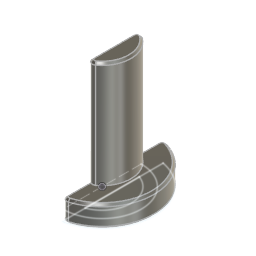
SpoolHanger (Autodesk Fusion 360 design; units mm, degrees)
Autodesk Fusion 360 part; units mm, degrees
note: some values were not read from the file. Chosen so that the rebuilt part matches the saved one: which face or edge a step refers to. Set by a fixed rule: which sketch regions a step uses.
sketch "Sketch1" plane through (0, 0, 0) normal (0, 0, 1) x (1, 0, 0) in component "VerticalArm"
  line L0 (0, 10.4) -> (0, -10.4)
  line L1 (0, 10.4) -> (-131.0205, 10.4)
  line L2 (0, -10.4) -> (-131.0205, -10.4)
  circle A0 centre (-150, 0) radius 21.6421
  line L3 (-139.8, -10.2) -> (-160.2, -10.2)
  line L4 (-160.2, -10.2) -> (-160.2, 10.2)
  line L5 (-160.2, 10.2) -> (-139.8, 10.2)
  line L6 (-139.8, 10.2) -> (-139.8, -10.2)
  line L7 (-139.8, -10.2) -> (-160.2, 10.2) construction
  line L8 (-160.2, -10.2) -> (-139.8, 10.2) construction
  line L9 (-150, 21.6421) -> (-150, -21.6421) construction
  line L10 (-150, 0) -> (0, 0) construction
  point P0 (-150, 0)
  dimension "d137" = 43.2843
  dimension "d138" = 20.4
  dimension "d253" = 20.8
  dimension "d255" = 150
  constraint coincident L10.end origin
  constraint vertical L0
  constraint perpendicular L0 L1
  constraint perpendicular L0 L2
  constraint equal L1 L2
  constraint horizontal L3
  constraint perpendicular L3 L4
  constraint parallel L3 L5
  constraint parallel L4 L6
  constraint coincident L7 P0
  constraint coincident L8 P0
  constraint coincident P0 A0.centre
  constraint equal L4 L5
  constraint midpoint L10.end L0
  constraint vertical L9
  constraint coincident P0 L9
  constraint coincident A0 L9.start
  constraint coincident A0 L9.end
  constraint perpendicular L0 L10
  constraint coincident A0 L1.end
  measures "d137" diameter of A0
  measures "d138" distance of L3.end L4.end
  measures "d253" distance of L0.start L0.end
  measures "d255" distance of L0 L9
sketch "Sketch1 (2)" plane through (0, 0, 0) normal (0, 0, 1) x (1, 0, 0) in component "HorizontalBarInnerPart"
  line L0 (80.8, -9.2) -> (-80.8, -9.2)
  line L1 (-80.8, -9.2) -> (-80.8, 9.2)
  line L2 (-80.8, 9.2) -> (80.8, 9.2)
  line L3 (80.8, 9.2) -> (80.8, -9.2)
  line L4 (80.8, -9.2) -> (-80.8, 9.2) construction
  line L5 (-80.8, -9.2) -> (80.8, 9.2) construction
  arc A0 (-80.8, 9.2) -> (-80.8, -9.2) centre (-80.8, 0) ccw
  arc A1 (-82.4, 7.4297) -> (-82.4, -7.4297) centre (-80.8, 0) ccw
  line L6 (-82.4, -7.4297) -> (-82.4, 7.4297)
  line L7 (0, 9.2) -> (0, -9.2)
  arc A2 (82.4, -7.4297) -> (82.4, 7.4297) centre (80.8, 0) ccw
  arc A3 (80.8, -9.2) -> (80.8, 9.2) centre (80.8, 0) ccw
  line L8 (82.4, -7.4297) -> (82.4, 7.4297)
  dimension "d81" = 161.6
  dimension "d82" = 18.4
  constraint horizontal L0
  constraint perpendicular L0 L1
  constraint parallel L0 L2
  constraint parallel L1 L3
  constraint coincident L4 origin
  constraint coincident L5 origin
  constraint tangent L0 A0
  constraint midpoint L2 L7.start
  constraint midpoint L0 L7.end
  constraint symmetric L0.end L7 L0.start
  constraint symmetric L1.end L7 L2.end
  constraint symmetric A0 L7 A3
  constraint symmetric A1.end L7 A2.start
  constraint symmetric A1.start L7 A2.end
  constraint symmetric A1 L7 A2
  measures "d81" distance of L1.end L2.end
  measures "d82" distance of L0.end L1.end
extrude "Extrude1" add sketch "Sketch1" along normal blind 20 makes body 1 in component "VerticalArm"
extrude "Extrude1'" add sketch "Sketch1 (2)" along normal blind 18.4 separate body makes body 2 in component "HorizontalBarInnerPart"
chamfer "Chamfer2" distance 1 angle 45 12 edges at (0, 9.2, 0) (90, 0, 0) (0, -9.2, 0) (-90, 0, 0) (0, 9.2, 18.4) (-90, 0, 18.4) (0, -9.2, 18.4) (90, 0, 18.4) (-82.4, 0, 18.4) (82.4, 0, 18.4) (82.4, 0, 0) (-82.4, 0, 0) on bodies 2 in component "HorizontalBarInnerPart"
sketch "Sketch1 (3)" plane through (0, 0, 0) normal (0, 0, 1) x (1, 0, 0) in component "HorizontalBarMiddlePart"
  circle A0 centre (0, 0) radius 14.425
  circle A1 centre (0, 0) radius 16.025
  line L0 (10.2, 10.2) -> (-10.2, 10.2)
  line L1 (-10.2, 10.2) -> (-10.2, -10.2)
  line L2 (-10.2, -10.2) -> (10.2, -10.2)
  line L3 (10.2, -10.2) -> (10.2, 10.2)
  line L4 (10.2, 10.2) -> (-10.2, -10.2) construction
  line L5 (-10.2, 10.2) -> (10.2, -10.2) construction
  line L6 (-8.297, 11.8) -> (8.297, 11.8)
  line L7 (0, 0) -> (0, 14.425) construction
  line L8 (-0.8, 11.8) -> (-0.8, 14.4028)
  line L9 (0.8, 11.8) -> (0.8, 14.4028)
  dimension "HorizontalBarOuterPartThickness" = 1.6
  dimension "d238" = 20.4
  dimension "d262" = 1.6
  dimension "d263" = 1.6
  constraint coincident A0.centre A1.centre
  constraint horizontal L0
  constraint perpendicular L0 L1
  constraint parallel L0 L2
  constraint parallel L1 L3
  constraint coincident L4 A0.centre
  constraint coincident L5 A0.centre
  constraint equal L2 L3
  constraint coincident A0 L1.end
  constraint horizontal L6
  constraint coincident A0 L6.start
  constraint coincident A0 L6.end
  constraint coincident A0 L7.end
  constraint perpendicular L6 L7
  constraint coincident L6 L8.start
  constraint coincident A0 L8.end
  constraint perpendicular L6 L8
  constraint coincident L6 L9.start
  constraint coincident A0 L9.end
  constraint perpendicular L6 L9
  constraint symmetric L7 L8 L9
  measures "d238" distance of L0.end L1.end
  measures "d262" distance of L0 L6
  measures "d263" distance of L8 L9
sketch "Sketch1 (4)" plane through (0, 0, 0) normal (0, 0, 1) x (1, 0, 0) in component "HorizontalBarPin"
  line L0 (0, 9.2) -> (0, -9.2) construction
  arc A0 (0, -9.2) -> (0, 9.2) centre (0, 0) ccw
  arc A1 (2.4, -6.3624) -> (2.4, 6.3624) centre (0, 0) ccw
  line L1 (2.4, 6.3624) -> (2.4, -6.3624)
  line L2 (2.4, 11.9616) -> (2.4, -11.9616)
  arc A2 (2.4, -11.9616) -> (2.4, 11.9616) centre (0, 0) ccw
  dimension "d280" = 18.4
  dimension "d282" = -2.4
  dimension "d283" = 3
  constraint midpoint A0.centre L0
  constraint vertical L0
  constraint coincident A0.centre A1.centre
  constraint vertical L2
  constraint collinear L1 L2
  measures "d280" distance of L0.start L0.end
  measures "d283" distance of A0 A2
extrude "Extrude1''" add sketch "Sketch1 (4)" along normal blind 5 separate body makes body 3 in component "HorizontalBarPin"
extrude "Extrude2" add sketch "Sketch1 (4)" along normal blind 30 contours A1 L1 L2 bodies 3 in component "HorizontalBarPin"
sketch "Sketch1 (5)" plane through (0, 0, 0) normal (0, 0, 1) x (1, 0, 0) in component "RailMount"
  line L0 (60, -8) -> (-60, -8)
  line L1 (-60, -8) -> (-60, 8)
  line L2 (-60, 8) -> (60, 8)
  line L3 (60, 8) -> (60, -8)
  line L4 (60, -8) -> (-60, 8) construction
  line L5 (-60, -8) -> (60, 8) construction
  line L6 (-60, 2.6667) -> (60, 2.6667) construction
  line L7 (-60, -2.6667) -> (60, -2.6667) construction
  line L8 (-52.5, 2.6667) -> (-27.5, 2.6667)
  line L9 (-52.5, 2.6667) -> (-47.5, -2.6667)
  line L10 (-32.5, -2.6667) -> (-7.5, -2.6667)
  line L11 (-32.5, -2.6667) -> (-27.5, 2.6667)
  line L12 (-12.5, 2.6667) -> (12.5, 2.6667)
  line L13 (-7.5, -2.6667) -> (-12.5, 2.6667)
  line L14 (7.5, -2.6667) -> (32.5, -2.6667)
  line L15 (7.5, -2.6667) -> (12.5, 2.6667)
  line L16 (27.5, 2.6667) -> (52.5, 2.6667)
  line L17 (32.5, -2.6667) -> (27.5, 2.6667)
  line L18 (-60, -2.6667) -> (-47.5, -2.6667)
  line L19 (47.5, -2.6667) -> (60, -2.6667)
  line L20 (52.5, 2.6667) -> (47.5, -2.6667)
  dimension "TotalRailThickness" = 16
  dimension "d164" = 5.3333
  dimension "d165" = 5.3333
  dimension "d171" = 12.5
  dimension "d172" = 25
  dimension "d174" = 120
  dimension "d227" = 46.848
  constraint horizontal L0
  constraint perpendicular L0 L1
  constraint parallel L0 L2
  constraint parallel L1 L3
  constraint coincident L4 origin
  constraint coincident L5 origin
  constraint coincident L1 L6.start
  constraint coincident L3 L6.end
  constraint perpendicular L3 L6
  constraint coincident L1 L7.start
  constraint coincident L3 L7.end
  constraint horizontal L7
  constraint coincident L7 L9.end
  constraint coincident L6 L8.start
  constraint coincident L6 L8.end
  constraint coincident L7 L10.start
  constraint parallel L7 L10
  constraint equal L9 L11
  constraint coincident L6 L12.start
  constraint coincident L6 L12.end
  constraint equal L9 L13
  constraint coincident L7 L14.start
  constraint coincident L7 L14.end
  constraint equal L9 L15
  constraint coincident L6 L16.start
  constraint coincident L6 L16.end
  constraint equal L9 L17
  constraint coincident L9.end L18.end
  constraint equal L8 L10
  constraint equal L8 L12
  constraint equal L8 L14
  constraint equal L8 L16
  constraint coincident L7 L19.start
  constraint coincident L7 L19.end
  constraint equal L18 L19
  constraint equal L9 L20
  constraint coincident L7.end L19.end
  constraint coincident L16.end L20.start
  measures "TotalRailThickness" distance of L0.end L1.end
  measures "d164" distance of L0 L7
  measures "d165" distance of L2 L6
  measures "d171" distance of L7.start L9.end
  measures "d172" distance of L8.start L8.end
  measures "d174" distance of L1.end L2.end
  measures "d227" angle of L7 L11
extrude "Extrude2'" add sketch "Sketch1 (5)" along normal blind 200 separate body contours L1 L2 L3 L8 L9 L10 L11 L12 L13 L14 L15 L16 L17 L18 L19 L20 makes body 4 in component "RailMount"
move_face "OffsetFaces2" offset -0.4 13 faces at (-55.8333, -2.6667, 133.3333) (-24.1667, -2.6667, 133.3333) (15.8333, -2.6667, 133.3333) (51.6667, -2.6667, 66.6667) (-9.1667, -0.8889, 66.6667) (-50.8333, 0.8889, 66.6667) (30.8333, -0.8889, 66.6667) (-30.8333, -0.8889, 66.6667) (9.1667, -0.8889, 66.6667) (50.8333, 0.8889, 66.6667) (35.8333, 2.6667, 133.3333) (-4.1667, 2.6667, 66.6667) (-44.1667, 2.6667, 66.6667) on bodies 4 in component "RailMount"
sketch "Sketch3" plane through (0, -2.2667, 0) normal (0, -1, 0) x (1, 0, 0) in component "RailMount"
  line L0 (-31.5767, 0) -> (-8.4233, 0)
  line L1 (-8.4233, 0) -> (-8.4233, 200)
  line L2 (-8.4233, 200) -> (-31.5767, 200)
  line L3 (-31.5767, 200) -> (-31.5767, 0)
  line L4 (8.4233, 0) -> (31.5767, 0)
  line L5 (31.5767, 0) -> (31.5767, 200)
  line L6 (31.5767, 200) -> (8.4233, 200)
  line L7 (8.4233, 200) -> (8.4233, 0)
  line L8 (-14.55, 182.05) -> (-25.45, 182.05)
  line L9 (-25.45, 182.05) -> (-25.45, 156.65)
  line L10 (-25.45, 156.65) -> (-14.55, 156.65)
  line L11 (-14.55, 156.65) -> (-14.55, 182.05)
  line L12 (-14.55, 182.05) -> (-25.45, 156.65) construction
  line L13 (-25.45, 182.05) -> (-14.55, 156.65) construction
  line L14 (-31.5767, 100) -> (31.5767, 100) construction
  line L15 (0, 100) -> (0, 0) construction
  line L16 (-14.55, 182.05) -> (-20, 187.5)
  line L17 (-20, 187.5) -> (-25.45, 182.05)
  circle A0 centre (-20, 169.35) radius 2.5
  line L18 (-20, 182.05) -> (-20, 156.65) construction
  line L19 (-20, 172.8855) -> (-21.7678, 171.1178)
  line L20 (-20, 172.8855) -> (-18.2322, 171.1178)
  line L21 (-25.45, 169.35) -> (-14.55, 169.35) construction
  line L22 (-20, 165.8145) -> (-18.2322, 167.5822)
  line L23 (-20, 165.8145) -> (-21.7678, 167.5822)
  line L24 (-14.55, 156.65) -> (-8.4233, 156.65) construction
  line L25 (-25.45, 156.65) -> (-31.5767, 156.65) construction
  line L26 (-20, 151.2) -> (-25.45, 156.65)
  line L27 (-14.55, 156.65) -> (-20, 151.2)
  point P0 (-20, 169.35)
  dimension "d181" = 25.4
  dimension "d186" = 45
  dimension "d187" = 12.5
  dimension "d194" = 5
  dimension "d219" = 10.9
  dimension "d221" = 90
  constraint horizontal L8
  constraint perpendicular L8 L9
  constraint parallel L8 L10
  constraint parallel L9 L11
  constraint coincident L12 P0
  constraint coincident L13 P0
  constraint midpoint L3 L14.start
  constraint midpoint L5 L14.end
  constraint midpoint L14 L15.start
  constraint coincident L15.end origin
  constraint equal L16 L17
  constraint coincident P0 A0.centre
  constraint midpoint L8 L18.start
  constraint midpoint L10 L18.end
  constraint coincident L18 L19.start
  constraint equal L19 L20
  constraint tangent A0 L19
  constraint coincident A0 L19.end
  constraint coincident A0 L20.end
  constraint midpoint L9 L21.start
  constraint midpoint L11 L21.end
  constraint symmetric L19.start L21 L22.start
  constraint symmetric L19.end L21 L23.end
  constraint symmetric L20.end L21 L22.end
  constraint coincident L1 L24.end
  constraint perpendicular L1 L24
  constraint coincident L3 L25.end
  constraint perpendicular L3 L25
  constraint equal L24 L25
  constraint symmetric L8.start L21 L10.end
  constraint symmetric L8.end L21 L9.end
  constraint symmetric L16.end L21 L26.start
  measures "d181" distance of L8.end L9.end
  measures "d186" angle of L8 L16
  measures "d187" distance of L2 L16.end
  measures "d194" diameter of A0
  measures "d219" distance of L8.start L8.end
  measures "d221" angle of L19 L20
ref_plane "WorkPlane1" through (0, 0, 100) normal (0, 0, 1) x (1, 0, 0) in component "RailMount"
extrude "Extrude3" cut sketch "Sketch3" against normal blind 3.9 contours L8 L9 L10 L11 | L8 L16 L17 | L10 L26 L27 | A0 | A0 L19 L20 | A0 L22 L23 bodies 4 in component "RailMount"
extrude "Extrude4" cut sketch "Sketch3" against normal through all contours A0 | A0 L19 L20 | A0 L22 L23 bodies 4 in component "RailMount"
mirror "Mirror1" about plane through (0, 0, 0) normal (1, 0, 0) of "Extrude3", "Extrude4" in component "RailMount"
mirror "Mirror3" about plane through (0, 0, 100) normal (0, 0, 1) of "Extrude3", "Extrude4" in component "RailMount"
mirror "Mirror4" about plane through (0, 0, 0) normal (1, 0, 0) of "Mirror3" in component "RailMount"
fillet "Fillet1" radius 0.5 48 edges at (48.4233, -2.2667, 100) (54.2116, -2.2667, 0) (60, -2.2667, 100) (54.2116, -2.2667, 200) (50.9233, 0.4, 200) (53.4233, 3.0667, 100) (50.9233, 0.4, 0) (40, 3.0667, 0) (29.0767, 0.4, 0) (20, -2.2667, 0) (10.9233, 0.4, 0) (0, 3.0667, 0) (-10.9233, 0.4, 0) (-20, -2.2667, 0) (-29.0767, 0.4, 0) (-40, 3.0667, 0) (-50.9233, 0.4, 0) (-54.2116, -2.2667, 0) (-60, 2.8667, 0) (0, 8, 0) (60, 2.8667, 0) (60, 2.8667, 200) (60, 8, 100) (40, 3.0667, 200) (29.0767, 0.4, 200) (20, -2.2667, 200) (10.9233, 0.4, 200) (0, 3.0667, 200) (-10.9233, 0.4, 200) (-20, -2.2667, 200) (-29.0767, 0.4, 200) (-40, 3.0667, 200) (-50.9233, 0.4, 200) (-54.2116, -2.2667, 200) (-60, 2.8667, 200) (0, 8, 200) (26.5767, 3.0667, 100) (31.5767, -2.2667, 100) (8.4233, -2.2667, 100) (13.4233, 3.0667, 100) (-13.4233, 3.0667, 100) (-8.4233, -2.2667, 100) (-31.5767, -2.2667, 100) (-26.5767, 3.0667, 100) (-53.4233, 3.0667, 100) (-48.4233, -2.2667, 100) (-60, -2.2667, 100) (-60, 8, 100) on bodies 4 in component "RailMount"
sketch "Sketch1 (6)" plane through (0, 0, 0) normal (0, 0, 1) x (1, 0, 0) in component "RailMountInsert"
  line L0 (5.05, -12.3) -> (-5.05, -12.3) construction
  line L1 (-5.05, -12.3) -> (-5.05, 12.3)
  line L2 (-5.05, 12.3) -> (5.05, 12.3) construction
  line L3 (5.05, 12.3) -> (5.05, -12.3)
  line L4 (5.05, -12.3) -> (-5.05, 12.3) construction
  line L5 (-5.05, -12.3) -> (5.05, 12.3) construction
  line L6 (-5.05, 12.3) -> (0, 17.35)
  line L7 (0, 17.35) -> (5.05, 12.3)
  line L8 (-5.05, -12.3) -> (0, -17.35)
  line L9 (0, -17.35) -> (5.05, -12.3)
  circle A0 centre (0, 0) radius 2.25
  dimension "d202" = 24.6
  dimension "d203" = 4.5
  dimension "d216" = 10.1
  dimension "d218" = 45
  constraint horizontal L0
  constraint perpendicular L0 L1
  constraint parallel L0 L2
  constraint parallel L1 L3
  constraint coincident L4 A0.centre
  constraint coincident L5 A0.centre
  constraint coincident A0.centre origin
  constraint equal L6 L7
  constraint equal L6 L8
  constraint equal L6 L9
  measures "d202" distance of L0.end L1.end
  measures "d203" diameter of A0
  measures "d216" distance of L0.start L0.end
  measures "d218" angle of L2 L6
extrude "Extrude1'''" add sketch "Sketch1 (6)" along normal blind 3.5 separate body makes body 5 in component "RailMountInsert"
fillet "Fillet1'" radius 1 6 edges at (0, -17.35, 1.75) (5.05, -12.3, 1.75) (-5.05, -12.3, 1.75) (-5.05, 12.3, 1.75) (0, 17.35, 1.75) (5.05, 12.3, 1.75) on bodies 5 in component "RailMountInsert"
chamfer "Chamfer1" distance 2 angle 45 1 edges at (-2.0977, 0.8136, 3.5) on bodies 5 in component "RailMountInsert"
chamfer "Chamfer2'" distance 0.5 angle 45 1 edges at (-2.0977, 0.8136, 0) on bodies 5 in component "RailMountInsert"
sketch "Sketch1 (7)" plane through (0, 0, 0) normal (0, 0, 1) x (1, 0, 0) in component "Mount (1)"
  line L0 (60, -8) -> (-60, -8)
  line L1 (-60, -8) -> (-60, 8)
  line L2 (-60, 8) -> (60, 8)
  line L3 (60, 8) -> (60, -8)
  line L4 (60, -8) -> (-60, 8) construction
  line L5 (-60, -8) -> (60, 8) construction
  line L6 (-60, 2.6667) -> (60, 2.6667) construction
  line L7 (-60, -2.6667) -> (60, -2.6667) construction
  line L8 (-52.5, 2.6667) -> (-27.5, 2.6667)
  line L9 (-52.5, 2.6667) -> (-47.5, -2.6667)
  line L10 (-32.5, -2.6667) -> (-7.5, -2.6667)
  line L11 (-32.5, -2.6667) -> (-27.5, 2.6667)
  line L12 (-12.5, 2.6667) -> (12.5, 2.6667)
  line L13 (-7.5, -2.6667) -> (-12.5, 2.6667)
  line L14 (7.5, -2.6667) -> (32.5, -2.6667)
  line L15 (7.5, -2.6667) -> (12.5, 2.6667)
  line L16 (27.5, 2.6667) -> (52.5, 2.6667)
  line L17 (32.5, -2.6667) -> (27.5, 2.6667)
  line L18 (-60, -2.6667) -> (-47.5, -2.6667)
  line L19 (47.5, -2.6667) -> (60, -2.6667)
  line L20 (52.5, 2.6667) -> (47.5, -2.6667)
  dimension "TotalRailThickness_1" = 16
  dimension "d164_1" = 5.3333
  dimension "d165_1" = 5.3333
  dimension "d171_1" = 12.5
  dimension "d172_1" = 25
  dimension "d174_1" = 120
  dimension "d227_1" = 46.848
  constraint horizontal L0
  constraint perpendicular L0 L1
  constraint parallel L0 L2
  constraint parallel L1 L3
  constraint coincident L4 origin
  constraint coincident L5 origin
  constraint coincident L1 L6.start
  constraint coincident L3 L6.end
  constraint perpendicular L3 L6
  constraint coincident L1 L7.start
  constraint coincident L3 L7.end
  constraint horizontal L7
  constraint coincident L7 L9.end
  constraint coincident L6 L8.start
  constraint coincident L6 L8.end
  constraint coincident L7 L10.start
  constraint parallel L7 L10
  constraint equal L9 L11
  constraint coincident L6 L12.start
  constraint coincident L6 L12.end
  constraint equal L9 L13
  constraint coincident L7 L14.start
  constraint coincident L7 L14.end
  constraint equal L9 L15
  constraint coincident L6 L16.start
  constraint coincident L6 L16.end
  constraint equal L9 L17
  constraint coincident L9.end L18.end
  constraint equal L8 L10
  constraint equal L8 L12
  constraint equal L8 L14
  constraint equal L8 L16
  constraint coincident L7 L19.start
  constraint coincident L7 L19.end
  constraint equal L18 L19
  constraint equal L9 L20
  constraint coincident L7.end L19.end
  constraint coincident L16.end L20.start
  measures "TotalRailThickness_1" distance of L0.end L1.end
  measures "d164_1" distance of L0 L7
  measures "d165_1" distance of L2 L6
  measures "d171_1" distance of L7.start L9.end
  measures "d172_1" distance of L8.start L8.end
  measures "d174_1" distance of L1.end L2.end
  measures "d227_1" angle of L7 L11
extrude "Extrude1''''" add sketch "Sketch1 (7)" along normal blind 120 separate body contours L0 L1 L3 L8 L9 L10 L11 L12 L13 L14 L15 L16 L17 L18 L19 L20 makes body 6 in component "Mount (1)"
move_face "OffsetFaces2'" offset -0.4 13 faces at (35.8333, 2.6667, 40) (-4.1667, 2.6667, 40) (-44.1667, 2.6667, 40) (-50.8333, 0.8889, 40) (-30.8333, -0.8889, 40) (9.1667, -0.8889, 40) (50.8333, 0.8889, 40) (-9.1667, -0.8889, 40) (30.8333, -0.8889, 40) (51.6667, -2.6667, 40) (15.8333, -2.6667, 40) (-24.1667, -2.6667, 40) (-55.8333, -2.6667, 40) on bodies 6 in component "Mount (1)"
fillet "Fillet2" radius 0.5 14 edges at (-60, -3.0667, 60) (60, -3.0667, 60) (-46.5767, -3.0667, 60) (-51.5767, 2.2667, 60) (-28.4233, 2.2667, 60) (-33.4233, -3.0667, 60) (-6.5767, -3.0667, 60) (-11.5767, 2.2667, 60) (11.5767, 2.2667, 60) (6.5767, -3.0667, 60) (33.4233, -3.0667, 60) (28.4233, 2.2667, 60) (51.5767, 2.2667, 60) (46.5767, -3.0667, 60) on bodies 6 in component "Mount (1)"
sketch "Sketch1 (8)" plane through (0, 0, 0) normal (0, 0, 1) x (1, 0, 0) in component "Mount_HorizontalBar"
  line L0 (60, -8) -> (-60, -8)
  line L1 (-60, -8) -> (-60, 8)
  line L2 (-60, 8) -> (60, 8)
  line L3 (60, 8) -> (60, -8)
  line L4 (60, -8) -> (-60, 8) construction
  line L5 (-60, -8) -> (60, 8) construction
  line L6 (-60, 2.6667) -> (60, 2.6667) construction
  line L7 (-60, -2.6667) -> (60, -2.6667) construction
  line L8 (-52.5, 2.6667) -> (-27.5, 2.6667)
  line L9 (-52.5, 2.6667) -> (-47.5, -2.6667)
  line L10 (-32.5, -2.6667) -> (-7.5, -2.6667)
  line L11 (-32.5, -2.6667) -> (-27.5, 2.6667)
  line L12 (-12.5, 2.6667) -> (12.5, 2.6667)
  line L13 (-7.5, -2.6667) -> (-12.5, 2.6667)
  line L14 (7.5, -2.6667) -> (32.5, -2.6667)
  line L15 (7.5, -2.6667) -> (12.5, 2.6667)
  line L16 (27.5, 2.6667) -> (52.5, 2.6667)
  line L17 (32.5, -2.6667) -> (27.5, 2.6667)
  line L18 (-60, -2.6667) -> (-47.5, -2.6667)
  line L19 (47.5, -2.6667) -> (60, -2.6667)
  line L20 (52.5, 2.6667) -> (47.5, -2.6667)
  dimension "TotalRailThickness_1_1" = 16
  dimension "d164_1_1" = 5.3333
  dimension "d165_1_1" = 5.3333
  dimension "d171_1_1" = 12.5
  dimension "d172_1_1" = 25
  dimension "d174_1_1" = 120
  dimension "d227_1_1" = 46.848
  constraint horizontal L0
  constraint perpendicular L0 L1
  constraint parallel L0 L2
  constraint parallel L1 L3
  constraint coincident L4 origin
  constraint coincident L5 origin
  constraint coincident L1 L6.start
  constraint coincident L3 L6.end
  constraint perpendicular L3 L6
  constraint coincident L1 L7.start
  constraint coincident L3 L7.end
  constraint horizontal L7
  constraint coincident L7 L9.end
  constraint coincident L6 L8.start
  constraint coincident L6 L8.end
  constraint coincident L7 L10.start
  constraint parallel L7 L10
  constraint equal L9 L11
  constraint coincident L6 L12.start
  constraint coincident L6 L12.end
  constraint equal L9 L13
  constraint coincident L7 L14.start
  constraint coincident L7 L14.end
  constraint equal L9 L15
  constraint coincident L6 L16.start
  constraint coincident L6 L16.end
  constraint equal L9 L17
  constraint coincident L9.end L18.end
  constraint equal L8 L10
  constraint equal L8 L12
  constraint equal L8 L14
  constraint equal L8 L16
  constraint coincident L7 L19.start
  constraint coincident L7 L19.end
  constraint equal L18 L19
  constraint equal L9 L20
  constraint coincident L7.end L19.end
  constraint coincident L16.end L20.start
  measures "TotalRailThickness_1_1" distance of L0.end L1.end
  measures "d164_1_1" distance of L0 L7
  measures "d165_1_1" distance of L2 L6
  measures "d171_1_1" distance of L7.start L9.end
  measures "d172_1_1" distance of L8.start L8.end
  measures "d174_1_1" distance of L1.end L2.end
  measures "d227_1_1" angle of L7 L11
extrude "Extrude1'''''" add sketch "Sketch1 (8)" along normal blind 20 separate body contours L0 L1 L3 L8 L9 L10 L11 L12 L13 L14 L15 L16 L17 L18 L19 L20 makes body 7 in component "Mount_HorizontalBar"
move_face "OffsetFaces2''" offset -0.4 13 faces at (-4.1667, 2.6667, 6.6667) (35.8333, 2.6667, 6.6667) (-44.1667, 2.6667, 13.3333) (-50.8333, 0.8889, 6.6667) (-30.8333, -0.8889, 6.6667) (9.1667, -0.8889, 6.6667) (50.8333, 0.8889, 6.6667) (-9.1667, -0.8889, 6.6667) (30.8333, -0.8889, 6.6667) (-24.1667, -2.6667, 6.6667) (15.8333, -2.6667, 6.6667) (51.6667, -2.6667, 6.6667) (-55.8333, -2.6667, 6.6667) on bodies 7 in component "Mount_HorizontalBar"
fillet "Fillet2'" radius 0.5 16 edges at (-60, -8, 10) (60, -8, 10) (-60, -3.0667, 10) (60, -3.0667, 10) (-46.5767, -3.0667, 10) (-51.5767, 2.2667, 10) (-28.4233, 2.2667, 10) (-33.4233, -3.0667, 10) (-6.5767, -3.0667, 10) (-11.5767, 2.2667, 10) (11.5767, 2.2667, 10) (6.5767, -3.0667, 10) (33.4233, -3.0667, 10) (28.4233, 2.2667, 10) (51.5767, 2.2667, 10) (46.5767, -3.0667, 10) on bodies 7 in component "Mount_HorizontalBar"
combine "Combine3" operation add target body 1 tool bodies 7 body 7 seen with x (0, -1, 0) y (1, 0, 0) z (0, 0, 1) at (8, 0, 0) keep tools in component "VerticalArm"
fillet "Fillet3" radius 25 2 edges at (0, 10.4, 10) (0, -10.4, 10) on bodies 1 in component "VerticalArm"
chamfer "Chamfer1'" distance 0.5 angle 45 83 edges at (-171.6421, 0, 20) (-171.6421, 0, 0) (-139.8, 0, 20) (-150, 10.2, 20) (-160.2, 0, 20) (-150, -10.2, 0) (-139.8, 0, 0) (-150, 10.2, 0) (-160.2, 0, 0) (-78.0102, -10.4, 0) (-78.0102, 10.4, 0) (-7.3223, 17.7223, 0) (0, 47.45, 0) (0.1464, 59.8536, 0) (2.4667, 60, 0) (4.7869, 59.8536, 0) (4.9333, 53.6154, 0) (5.2346, 47.272, 0) (7.6, 49.0767, 0) (9.9654, 50.8814, 0) (10.2667, 40, 0) (9.9654, 29.1186, 0) (7.6, 30.9233, 0) (5.2346, 32.728, 0) (4.9333, 20, 0) (5.2346, 7.272, 0) (7.6, 9.0767, 0) (9.9654, 10.8814, 0) (10.2667, 0, 0) (9.9654, -10.8814, 0) (7.6, -9.0767, 0) (5.2346, -7.272, 0) (4.9333, -20, 0) (5.2346, -32.728, 0) (7.6, -30.9233, 0) (9.9654, -29.1186, 0) (10.2667, -40, 0) (9.9654, -50.8814, 0) (7.6, -49.0767, 0) (5.2346, -47.272, 0) (4.9333, -53.6154, 0) (4.7869, -59.8536, 0) (2.4667, -60, 0) (0.1464, -59.8536, 0) (0, -47.45, 0) (-7.3223, -17.7223, 0) (-78.0102, -10.4, 20) (-7.3223, -17.7223, 20) (0, -47.45, 20) (0.1464, -59.8536, 20) (2.4667, -60, 20) (4.7869, -59.8536, 20) (4.9333, -53.6154, 20) (5.2346, -47.272, 20) (7.6, -49.0767, 20) (9.9654, -50.8814, 20) (10.2667, -40, 20) (9.9654, -29.1186, 20) (7.6, -30.9233, 20) (5.2346, -32.728, 20) (4.9333, -20, 20) (5.2346, -7.272, 20) (7.6, -9.0767, 20) (9.9654, -10.8814, 20) (10.2667, 0, 20) (9.9654, 10.8814, 20) (7.6, 9.0767, 20) (5.2346, 7.272, 20) (4.9333, 20, 20) (5.2346, 32.728, 20) (7.6, 30.9233, 20) (9.9654, 29.1186, 20) (10.2667, 40, 20) (9.9654, 50.8814, 20) (7.6, 49.0767, 20) (5.2346, 47.272, 20) (4.9333, 53.6154, 20) (4.7869, 59.8536, 20) (2.4667, 60, 20) (0.1464, 59.8536, 20) (0, 47.45, 20) (-7.3223, 17.7223, 20) (-78.0102, 10.4, 20) on bodies 1 in component "VerticalArm"
extrude "Extrude3'" add sketch "Sketch1 (3)" along normal blind 120 separate body makes body 8 in component "HorizontalBarMiddlePart"
sketch "Sketch1 (9)" plane through (0, 0, 0) normal (0, 0, 1) x (1, 0, 0) in component "HorizontalBarOuterPart"
  circle A0 centre (0, 0) radius 16.7584
  circle A1 centre (0, 0) radius 25.8
  circle A2 centre (0, 0) radius 24.2
  line L0 (11.85, 11.85) -> (-11.85, 11.85) construction
  line L1 (-11.85, 11.85) -> (-11.85, -11.85) construction
  line L2 (-11.85, -11.85) -> (11.85, -11.85) construction
  line L3 (11.85, -11.85) -> (11.85, 11.85) construction
  line L4 (11.85, 11.85) -> (-11.85, -11.85) construction
  line L5 (-11.85, 11.85) -> (11.85, -11.85) construction
  circle A3 centre (0, 0) radius 18.3584
  line L6 (0, 0) -> (24.2, 0) construction
  line L7 (18.341, 0.8) -> (24.1868, 0.8)
  line L8 (18.341, -0.8) -> (24.1868, -0.8)
  dimension "d125_1" = 51.6
  dimension "d238_1" = 23.7
  dimension "d257" = 1.6
  dimension "d259" = 1.6
  constraint horizontal L0
  constraint perpendicular L0 L1
  constraint parallel L0 L2
  constraint parallel L1 L3
  constraint coincident L4 A0.centre
  constraint coincident L5 A0.centre
  constraint coincident A0.centre A1.centre
  constraint equal L2 L3
  constraint concentric A0 A2
  constraint coincident A0 L0.start
  constraint coincident A2 L6.end
  constraint horizontal L6
  constraint coincident A3 L7.start
  constraint coincident A2 L7.end
  constraint parallel L6 L7
  constraint coincident A3 L8.start
  constraint coincident A2 L8.end
  constraint horizontal L8
  constraint symmetric L6 L7 L8
  measures "d125_1" diameter of A1
  measures "d238_1" distance of L0.end L1.end
  measures "d259" distance of L7 L8
extrude "Extrude3''" add sketch "Sketch1 (9)" along normal blind 120 separate body contours A1 | A3 makes body 9 at (25.6718, -2.5689, 80) makes body 10 at (18.2672, -1.8279, 40) in component "HorizontalBarOuterPart"
extrude "Extrude4'" add sketch "Sketch1 (9)" along normal blind 120 separate body contours A2 A3 L7 L8 picked at (20.3004, -0.4445) makes body 11 in component "HorizontalBarOuterPart"
pattern_circular "C-Pattern3" count 12 over 360 about axis through (0, 0, 1.75) along (0, 0, 1) of bodies 11 makes body 12 at (17.1713, 10.8376, 40) makes body 13 at (10.8376, 17.1713, 40) makes body 14 at (0.8, 20.2896, 40) makes body 15 at (-10.8376, 17.1713, 40) makes body 16 at (-17.1713, 10.8376, 40) makes body 17 at (-20.2896, 0.8, 40) makes body 18 at (-17.9713, -9.452, 40) makes body 19 at (-9.452, -17.9713, 40) makes body 20 at (-0.8, -20.2896, 40) makes body 21 at (10.8376, -17.1713, 40) makes body 22 at (17.9713, -9.452, 40) in component "HorizontalBarOuterPart"
combine "Combine3'" operation add target body 9 tool bodies 18 15 11 17 21 14 19 22 16 12 10 13 20 keep tools in component "HorizontalBarOuterPart"
extrude "Extrude6" add sketch "Sketch1 (3)" along normal blind 120 separate body contours A0 L0 L6 | A0 L6 L8 L9 makes body 23 in component "HorizontalBarMiddlePart"
pattern_circular "C-Pattern3'" count 4 over 360 about axis through (0, 0, 1.75) along (0, 0, 1) of bodies 23 makes body 24 at (-10.2, -3.4, 80) makes body 25 at (3.4, -10.2, 80) makes body 26 at (10.2, 3.4, 80) in component "HorizontalBarMiddlePart"
combine "Combine3''" operation add target body 8 tool bodies 23 24 25 26 keep tools in component "HorizontalBarMiddlePart"
fillet "Fillet2''" radius 1 4 edges at (2.4, -11.9616, 2.5) (2.4, -6.3624, 17.5) (2.4, 6.3624, 17.5) (2.4, 11.9616, 2.5) on bodies 3 in component "HorizontalBarPin"
chamfer "Chamfer2''" distance 0.5 angle 45 5 edges at (12.2, 0, 5) (2.8099, 11.4788, 5) (2.4, 7.6852, 5) (2.4, -7.6852, 5) (2.8099, -11.4788, 5) 2 faces at (5.6555, 0.3017, 0) (3.8607, 0.1645, 30) on bodies 3 in component "HorizontalBarPin"
component "VerticalArm" placed x (0, 1, 0) y (-1, 0, 0) z (0, 0, 1) at (0, -8, 0)
component "HorizontalBarInnerPart" placed x (1, 0, 0) y (0, 1, 0) z (0, 0, 1) at (0, 0, 0)
component "HorizontalBarMiddlePart" placed x (1, 0, 0) y (0, 1, 0) z (0, 0, 1) at (0, 0, 0)
component "HorizontalBarPin" placed x (1, 0, 0) y (0, 1, 0) z (0, 0, 1) at (0, 0, 0)
component "RailMount" placed x (1, 0, 0) y (0, 1, 0) z (0, 0, 1) at (0, 0, 0)
component "RailMountInsert" placed x (1, 0, 0) y (0, 1, 0) z (0, 0, 1) at (0, 0, 0)
component "Mount (1)" placed x (1, 0, 0) y (0, 1, 0) z (0, 0, 1) at (0, 0, 0)
component "Mount_HorizontalBar" placed x (1, 0, 0) y (0, 1, 0) z (0, 0, 1) at (0, 0, 0)
component "HorizontalBarOuterPart" placed x (1, 0, 0) y (0, 1, 0) z (0, 0, 1) at (0, 0, 0)
hidden bodies 23 24 25 26 10 11 12 13 14 15 16 17 18 19 20 21 22
equation "mountBaseNeckOuterEdge = 20 mm"
equation "mountBaseNeckChamfer = 2 mm"
equation "PrinterOffset = 0.4 mm"
equation "d65 = mountBaseNeckOuterEdge"
equation "d81 = SpoolWidth + 2 * mountBaseNeckOuterEdge + 4 * PrinterOffset"
equation "d82 = HorizontalBarThickness - 4 * PrinterOffset"
equation "d84 = HorizontalBarThickness - 4 * PrinterOffset"
equation "d87 = -HorizontalBarPinLoopThickness"
equation "HorizontalBarOuterPartThickness = HorizontalBarOuterPartThickness_"
equation "HorizontalBarWidth = 120 mm"
equation "d137 = mountBaseNeckOuterEdge * sqrt(2) + 15 mm"
equation "d138 = HorizontalBarThickness + PrinterOffset"
equation "d155 = HorizontalBarThickness + 10 mm"
equation "SpoolWidth = 120 mm"
equation "SpoolInnerDiameter = 52 mm"
equation "RailWidth = 65 mm"
equation "d164 = TotalRailThickness / 3"
equation "d165 = TotalRailThickness / 3"
equation "MountRailEdge = 25 mm"
equation "d171 = MountRailEdge / 2"
equation "d172 = MountRailEdge"
equation "d181 = MountRailEdge + PrinterOffset"
equation "d182 = -3.5 mm - PrinterOffset"
equation "d187 = MountRailEdge / 2"
equation "d202 = MountRailEdge - PrinterOffset"
equation "d216 = MountRailEdge / 2 - PrinterOffset - 2 mm"
equation "d219 = MountRailEdge / 2 + PrinterOffset - 2 mm"
equation "d164_1 = TotalRailThickness_1 / 3"
equation "d165_1 = TotalRailThickness_1 / 3"
equation "d171_1 = MountRailEdge / 2"
equation "d172_1 = MountRailEdge"
equation "d164_1_1 = TotalRailThickness_1_1 / 3"
equation "d165_1_1 = TotalRailThickness_1_1 / 3"
equation "d171_1_1 = MountRailEdge / 2"
equation "d172_1_1 = MountRailEdge"
equation "d175_1_1 = mountBaseNeckOuterEdge"
equation "SpoolRadius = 140 mm"
equation "d238 = HorizontalBarThickness + PrinterOffset"
equation "d240 = SpoolWidth"
equation "d250 = -RailMountOffset"
equation "d251 = -RailMountOffset"
equation "HorizontalBarOuterPartThickness_1 = 1.6 mm"
equation "d125_1 = SpoolInnerDiameter - PrinterOffset"
equation "d126_1 = -HorizontalBarOuterPartThickness_"
equation "d238_1 = HorizontalBarThickness + HorizontalBarOuterPartThickness_ + 4 * PrinterOffset + 0.5 mm"
equation "d240_1 = SpoolWidth"
equation "d242_1 = SpoolWidth"
equation "HorizontalBarThickness = 20 mm"
equation "d253 = mountBaseNeckOuterEdge + 2 * PrinterOffset"
equation "d255 = SpoolRadius + 10 mm"
equation "HorizontalBarOuterPartThickness_ = 1.6 mm"
equation "d257 = HorizontalBarOuterPartThickness_"
equation "d259 = HorizontalBarOuterPartThickness_"
equation "d262 = HorizontalBarOuterPartThickness_"
equation "d263 = HorizontalBarOuterPartThickness_"
equation "d264 = SpoolWidth"
equation "HorizontalBarPinLoopThickness = 1.6 mm"
equation "d278 = -RailMountOffset"
equation "RailMountOffset = PrinterOffset"
equation "d280 = HorizontalBarThickness - 4 * PrinterOffset"
equation "d282 = -HorizontalBarPinLoopThickness - 2 * PrinterOffset"
